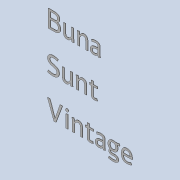
# Autodesk Inventor part: Vintage
Saved by Autodesk Inventor 2020 (Build 240168000, 168)
## iProperties
Created: 2021-01-22
Part Number: Vintage
Material: Generic
Document SubType Name: Modeling
Designer: Iulian Bors
Density: 1 g/cm^3
Appearance: Default
Author: Iulian Bors
Autodesk Inventor part; units mm, degrees
ref_plane "YZ Plane" through (0, 0, 0) normal (1, 0, 0) x (0, 1, 0)
ref_plane "XZ Plane" through (0, 0, 0) normal (0, 1, 0) x (-1, 0, 0)
ref_plane "XY Plane" through (0, 0, 0) normal (0, 0, 1) x (1, 0, 0)
sketch "Sketch1" plane through (0, 0, 0) normal (0, 0, 1) x (1, 0, 0)
  line L0 (-100, 150) -> (100, 150)
  line L1 (100, 150) -> (100, -150)
  line L2 (100, -150) -> (-100, -150)
  line L3 (-100, -150) -> (-100, 150)
  line L4 (-49.0032, 86.8855) -> (-35.0797, 86.8855) construction
  line L5 (-35.0797, 86.8855) -> (-35.0797, 72.9361) construction
  line L6 (-35.0797, 72.9361) -> (-49.0032, 72.9361) construction
  line L7 (-49.0032, 72.9361) -> (-49.0032, 86.8855) construction
  spline S0 degree 2 poles (-38.0317, 86.8855) (-36.2544, 86.8855) (-33.1501, 86.3405) (-30.8042, 84.9898) (-29.4535, 82.6675) (-29.4535, 80.8428) knots 0 0 0 1 2 3 4 4 4
  spline S1 degree 2 poles (-29.4535, 80.8428) (-29.4535, 79.7765) (-29.9511, 78.094) (-30.8279, 76.8144) (-32.1075, 75.8902) (-32.8895, 75.5822) knots 0 0 0 1 2 3 4 4 4
  line L8 (-32.8895, 75.5822) -> (-32.8895, 75.5348)
  spline S2 degree 2 poles (-32.8895, 75.5348) (-31.9416, 75.2978) (-30.1881, 74.2789) (-28.861, 72.7149) (-28.079, 70.5822) (-28.079, 69.2315) knots 0 0 0 1 2 3 4 4 4
  spline S3 degree 2 poles (-28.079, 69.2315) (-28.079, 67.2646) (-29.4772, 64.4684) (-31.9179, 62.6912) (-35.2354, 61.8618) (-37.1786, 61.8618) knots 0 0 0 1 2 3 4 4 4
  line L9 (-37.1786, 61.8618) -> (-45.899, 61.8618)
  line L10 (-45.899, 61.8618) -> (-45.899, 86.8855)
  line L11 (-45.899, 86.8855) -> (-38.0317, 86.8855)
  spline S4 degree 2 poles (-37.1786, 64.3973) (-35.9463, 64.3973) (-33.8136, 65.0135) (-32.2497, 66.2457) (-31.3492, 68.0466) (-31.3492, 69.2315) knots 0 0 0 1 2 3 4 4 4
  spline S5 degree 2 poles (-31.3492, 69.2315) (-31.3492, 70.4163) (-32.2497, 72.2172) (-33.8136, 73.4495) (-35.9463, 74.0656) (-37.1786, 74.0656) knots 0 0 0 1 2 3 4 4 4
  line L12 (-37.1786, 74.0656) -> (-42.6288, 74.0656)
  line L13 (-42.6288, 74.0656) -> (-42.6288, 64.3973)
  line L14 (-42.6288, 64.3973) -> (-37.1786, 64.3973)
  spline S6 degree 2 poles (-38.079, 76.6011) (-36.8231, 76.6011) (-34.8326, 77.0277) (-33.4819, 78.0229) (-32.7236, 79.658) (-32.7236, 80.8902) knots 0 0 0 1 2 3 4 4 4
  spline S7 degree 2 poles (-32.7236, 80.8902) (-32.7236, 81.9329) (-33.6004, 83.2836) (-34.335, 83.6627) knots 0 0 0 1 2 2 2
  spline S8 degree 2 poles (-34.335, 83.6627) (-35.0933, 84.0656) (-37.0364, 84.3499) (-38.079, 84.3499) knots 0 0 0 1 2 2 2
  line L15 (-38.079, 84.3499) -> (-42.6288, 84.3499)
  line L16 (-42.6288, 84.3499) -> (-42.6288, 76.6011)
  line L17 (-42.6288, 76.6011) -> (-38.079, 76.6011)
  line L18 (-8.5767, 62.1699) -> (-11.4677, 61.53)
  spline S9 degree 2 poles (-11.4677, 61.53) (-11.7994, 62.5727) (-11.9179, 63.5443) knots 0 0 0 1 1 1
  spline S10 degree 2 poles (-11.9179, 63.5443) (-11.989, 63.9945) (-12.1075, 65.3926) knots 0 0 0 1 1 1
  line L19 (-12.1075, 65.3926) -> (-12.4629, 65.3926)
  spline S11 degree 2 poles (-12.4629, 65.3926) (-13.4345, 63.639) (-14.8326, 62.5964) knots 0 0 0 1 1 1
  spline S12 degree 2 poles (-14.8326, 62.5964) (-16.3729, 61.4353) (-18.1027, 61.4353) knots 0 0 0 1 1 1
  spline S13 degree 2 poles (-18.1027, 61.4353) (-20.6857, 61.4353) (-22.0364, 62.6912) knots 0 0 0 1 1 1
  spline S14 degree 2 poles (-22.0364, 62.6912) (-23.1975, 63.7575) (-23.6715, 65.9376) knots 0 0 0 1 1 1
  spline S15 degree 2 poles (-23.6715, 65.9376) (-23.9558, 67.4542) (-23.9558, 70.4163) knots 0 0 0 1 1 1
  line L20 (-23.9558, 70.4163) -> (-23.9558, 79.9661)
  line L21 (-23.9558, 79.9661) -> (-20.97, 79.9661)
  line L22 (-20.97, 79.9661) -> (-20.97, 69.5632)
  spline S16 degree 2 poles (-20.97, 69.5632) (-20.97, 66.9803) (-20.4724, 65.8665) knots 0 0 0 1 1 1
  spline S17 degree 2 poles (-20.4724, 65.8665) (-19.7141, 64.2078) (-17.4629, 64.2078) knots 0 0 0 1 1 1
  spline S18 degree 2 poles (-17.4629, 64.2078) (-15.8516, 64.2078) (-14.335, 65.748) knots 0 0 0 1 1 1
  spline S19 degree 2 poles (-14.335, 65.748) (-13.2923, 66.767) (-12.1312, 68.7575) knots 0 0 0 1 1 1
  line L23 (-12.1312, 68.7575) -> (-12.1312, 79.9661)
  line L24 (-12.1312, 79.9661) -> (-9.1454, 79.9661)
  line L25 (-9.1454, 79.9661) -> (-9.1454, 68.7812)
  spline S20 degree 2 poles (-9.1454, 68.7812) (-9.1454, 66.4589) (-9.0269, 64.7528) knots 0 0 0 1 1 1
  spline S21 degree 2 poles (-9.0269, 64.7528) (-8.9558, 63.7101) (-8.5767, 62.1699) knots 0 0 0 1 1 1
  line L26 (-3.9558, 79.658) -> (-1.0885, 80.2978)
  spline S22 degree 2 poles (-1.0885, 80.2978) (-0.7568, 79.2552) (-0.6146, 78.2836) knots 0 0 0 1 1 1
  spline S23 degree 2 poles (-0.6146, 78.2836) (-0.5435, 77.8097) (-0.425, 76.4116) knots 0 0 0 1 1 1
  line L27 (-0.425, 76.4116) -> (-0.0696, 76.4116)
  spline S24 degree 2 poles (-0.0696, 76.4116) (0.8783, 78.1651) (2.3001, 79.2315) knots 0 0 0 1 1 1
  spline S25 degree 2 poles (2.3001, 79.2315) (3.8404, 80.3689) (5.5702, 80.3689) knots 0 0 0 1 1 1
  spline S26 degree 2 poles (5.5702, 80.3689) (8.1769, 80.3689) (9.5276, 79.113) knots 0 0 0 1 1 1
  spline S27 degree 2 poles (9.5276, 79.113) (10.6887, 78.0466) (11.1627, 75.8665) knots 0 0 0 1 1 1
  spline S28 degree 2 poles (11.1627, 75.8665) (11.447, 74.3736) (11.447, 71.4116) knots 0 0 0 1 1 1
  line L28 (11.447, 71.4116) -> (11.447, 61.8618)
  line L29 (11.447, 61.8618) -> (8.4612, 61.8618)
  line L30 (8.4612, 61.8618) -> (8.4612, 72.2409)
  spline S29 degree 2 poles (8.4612, 72.2409) (8.4612, 74.8239) (7.9636, 75.9376) knots 0 0 0 1 1 1
  spline S30 degree 2 poles (7.9636, 75.9376) (7.2053, 77.5964) (4.9304, 77.5964) knots 0 0 0 1 1 1
  spline S31 degree 2 poles (4.9304, 77.5964) (3.3428, 77.5964) (1.8025, 76.0561) knots 0 0 0 1 1 1
  spline S32 degree 2 poles (1.8025, 76.0561) (0.7598, 75.0371) (-0.4013, 73.0466) knots 0 0 0 1 1 1
  line L31 (-0.4013, 73.0466) -> (-0.4013, 61.8618)
  line L32 (-0.4013, 61.8618) -> (-3.3871, 61.8618)
  line L33 (-3.3871, 61.8618) -> (-3.3871, 72.9992)
  spline S33 degree 2 poles (-3.3871, 72.9992) (-3.3871, 75.3452) (-3.5056, 77.0514) knots 0 0 0 1 1 1
  spline S34 degree 2 poles (-3.5056, 77.0514) (-3.5767, 78.1177) (-3.9558, 79.658) knots 0 0 0 1 1 1
  line L34 (17.6319, 76.767) -> (16.8736, 79.2078)
  spline S35 degree 2 poles (16.8736, 79.2078) (19.7883, 80.3689) (22.9873, 80.3689) knots 0 0 0 1 1 1
  spline S36 degree 2 poles (22.9873, 80.3689) (25.7835, 80.3689) (27.2764, 79.421) knots 0 0 0 1 1 1
  spline S37 degree 2 poles (27.2764, 79.421) (28.9589, 78.3547) (28.9589, 75.748) knots 0 0 0 1 1 1
  line L35 (28.9589, 75.748) -> (28.9589, 68.639)
  spline S38 degree 2 poles (28.9589, 68.639) (28.9589, 67.1935) (28.9826, 65.7007) knots 0 0 0 1 1 1
  spline S39 degree 2 poles (28.9826, 65.7007) (29.0063, 64.8239) (29.1721, 63.8523) knots 0 0 0 1 1 1
  spline S40 degree 2 poles (29.1721, 63.8523) (29.2906, 62.9518) (29.5276, 62.1225) knots 0 0 0 1 1 1
  line L36 (29.5276, 62.1225) -> (26.684, 61.5063)
  spline S41 degree 2 poles (26.684, 61.5063) (26.2811, 62.6675) (26.1627, 64.113) knots 0 0 0 1 1 1
  line L37 (26.1627, 64.113) -> (25.8309, 64.1604)
  spline S42 degree 2 poles (25.8309, 64.1604) (23.6745, 61.4353) (20.3333, 61.4353) knots 0 0 0 1 1 1
  spline S43 degree 2 poles (20.3333, 61.4353) (17.8925, 61.4353) (14.9304, 64.1367) (14.9304, 66.6011) knots 0 0 0 1 2 2 2
  spline S44 degree 2 poles (14.9304, 66.6011) (14.9304, 68.4258) (16.5418, 70.7717) (18.0347, 71.5537) knots 0 0 0 1 2 2 2
  spline S45 degree 2 poles (18.0347, 71.5537) (20.357, 72.8334) (24.5513, 72.8334) knots 0 0 0 1 1 1
  spline S46 degree 2 poles (24.5513, 72.8334) (25.12, 72.8334) (26.0442, 72.8097) knots 0 0 0 1 1 1
  line L38 (26.0442, 72.8097) -> (26.0442, 75.44)
  spline S47 degree 2 poles (26.0442, 75.44) (26.0442, 76.6959) (24.5276, 77.8097) (22.8925, 77.8097) knots 0 0 0 1 2 2 2
  spline S48 degree 2 poles (22.8925, 77.8097) (20.4992, 77.8097) (17.6319, 76.767) knots 0 0 0 1 1 1
  line L39 (26.0442, 66.9329) -> (26.0442, 70.6059)
  spline S49 degree 2 poles (26.0442, 70.6059) (25.5702, 70.6296) (24.6698, 70.6296) knots 0 0 0 1 1 1
  spline S50 degree 2 poles (24.6698, 70.6296) (23.1532, 70.6296) (21.8499, 70.3689) knots 0 0 0 1 1 1
  spline S51 degree 2 poles (21.8499, 70.3689) (19.9541, 69.9898) (17.8451, 68.331) (17.8451, 66.7907) knots 0 0 0 1 2 2 2
  spline S52 degree 2 poles (17.8451, 66.7907) (17.8451, 63.9945) (20.8783, 63.9945) knots 0 0 0 1 1 1
  spline S53 degree 2 poles (20.8783, 63.9945) (22.4423, 63.9945) (23.793, 64.8239) knots 0 0 0 1 1 1
  spline S54 degree 2 poles (23.793, 64.8239) (24.9067, 65.5348) (26.0442, 66.9329) knots 0 0 0 1 1 1
  spline S55 degree 2 poles (-45.97, 9.0243) (-45.2591, 8.74) (-43.6715, 8.2661) (-42.0127, 7.9106) (-40.3539, 7.6973) (-39.5482, 7.6973) knots 0 0 0 1 2 3 4 4 4
  spline S56 degree 2 poles (-39.5482, 7.6973) (-38.1738, 7.6973) (-35.9463, 8.3134) (-34.3587, 9.522) (-33.4819, 11.2755) (-33.4819, 12.413) knots 0 0 0 1 2 3 4 4 4
  spline S57 degree 2 poles (-33.4819, 12.413) (-33.4819, 13.5504) (-34.2876, 14.9959) (-35.8279, 15.9675) (-38.1027, 16.6547) (-39.5482, 17.0101) knots 0 0 0 1 2 3 4 4 4
  spline S58 degree 2 poles (-39.5482, 17.0101) (-41.1596, 17.413) (-43.8373, 18.4556) (-45.8042, 20.0907) (-46.9179, 22.5078) (-46.9179, 24.3324) knots 0 0 0 1 2 3 4 4 4
  spline S59 degree 2 poles (-46.9179, 24.3324) (-46.9179, 25.8016) (-45.7331, 28.195) (-43.5767, 29.9011) (-40.5672, 30.8016) (-38.7189, 30.8016) knots 0 0 0 1 2 3 4 4 4
  spline S60 degree 2 poles (-38.7189, 30.8016) (-37.8421, 30.8016) (-35.9937, 30.5646) (-34.1928, 30.1855) (-32.4392, 29.6405) (-31.6809, 29.3087) knots 0 0 0 1 2 3 4 4 4
  line L40 (-31.6809, 29.3087) -> (-32.7236, 26.7258)
  spline S61 degree 2 poles (-32.7236, 26.7258) (-33.3634, 26.9864) (-34.6667, 27.4604) (-36.1122, 27.8395) (-37.771, 28.0765) (-38.7189, 28.0765) knots 0 0 0 1 2 3 4 4 4
  spline S62 degree 2 poles (-38.7189, 28.0765) (-39.6904, 28.0765) (-41.4203, 27.6499) (-42.771, 26.7732) (-43.553, 25.3514) (-43.553, 24.3324) knots 0 0 0 1 2 3 4 4 4
  spline S63 degree 2 poles (-43.553, 24.3324) (-43.553, 23.195) (-42.7473, 21.7495) (-41.207, 20.7779) (-38.9321, 20.0907) (-37.4866, 19.7352) knots 0 0 0 1 2 3 4 4 4
  spline S64 degree 2 poles (-37.4866, 19.7352) (-35.899, 19.3087) (-33.1975, 18.2898) (-31.2307, 16.6547) (-30.117, 14.2139) (-30.117, 12.413) knots 0 0 0 1 2 3 4 4 4
  spline S65 degree 2 poles (-30.117, 12.413) (-30.117, 10.5172) (-31.5151, 7.721) (-34.0506, 5.8727) (-37.5103, 4.9722) (-39.5482, 4.9722) knots 0 0 0 1 2 3 4 4 4
  spline S66 degree 2 poles (-39.5482, 4.9722) (-43.3871, 4.9722) (-47.0127, 6.4414) knots 0 0 0 1 1 1
  line L41 (-47.0127, 6.4414) -> (-45.97, 9.0243)
  line L42 (-10.3302, 5.7068) -> (-13.2212, 5.067)
  spline S67 degree 2 poles (-13.2212, 5.067) (-13.553, 6.1097) (-13.6715, 7.0812) knots 0 0 0 1 1 1
  spline S68 degree 2 poles (-13.6715, 7.0812) (-13.7426, 7.5315) (-13.861, 8.9296) knots 0 0 0 1 1 1
  line L43 (-13.861, 8.9296) -> (-14.2165, 8.9296)
  spline S69 degree 2 poles (-14.2165, 8.9296) (-15.1881, 7.176) (-16.5862, 6.1334) knots 0 0 0 1 1 1
  spline S70 degree 2 poles (-16.5862, 6.1334) (-18.1264, 4.9722) (-19.8563, 4.9722) knots 0 0 0 1 1 1
  spline S71 degree 2 poles (-19.8563, 4.9722) (-22.4392, 4.9722) (-23.7899, 6.2281) knots 0 0 0 1 1 1
  spline S72 degree 2 poles (-23.7899, 6.2281) (-24.9511, 7.2945) (-25.425, 9.4746) knots 0 0 0 1 1 1
  spline S73 degree 2 poles (-25.425, 9.4746) (-25.7094, 10.9912) (-25.7094, 13.9533) knots 0 0 0 1 1 1
  line L44 (-25.7094, 13.9533) -> (-25.7094, 23.503)
  line L45 (-25.7094, 23.503) -> (-22.7236, 23.503)
  line L46 (-22.7236, 23.503) -> (-22.7236, 13.1002)
  spline S74 degree 2 poles (-22.7236, 13.1002) (-22.7236, 10.5172) (-22.226, 9.4035) knots 0 0 0 1 1 1
  spline S75 degree 2 poles (-22.226, 9.4035) (-21.4677, 7.7447) (-19.2165, 7.7447) knots 0 0 0 1 1 1
  spline S76 degree 2 poles (-19.2165, 7.7447) (-17.6051, 7.7447) (-16.0885, 9.285) knots 0 0 0 1 1 1
  spline S77 degree 2 poles (-16.0885, 9.285) (-15.0459, 10.304) (-13.8847, 12.2945) knots 0 0 0 1 1 1
  line L47 (-13.8847, 12.2945) -> (-13.8847, 23.503)
  line L48 (-13.8847, 23.503) -> (-10.899, 23.503)
  line L49 (-10.899, 23.503) -> (-10.899, 12.3182)
  spline S78 degree 2 poles (-10.899, 12.3182) (-10.899, 9.9959) (-10.7805, 8.2898) knots 0 0 0 1 1 1
  spline S79 degree 2 poles (-10.7805, 8.2898) (-10.7094, 7.2471) (-10.3302, 5.7068) knots 0 0 0 1 1 1
  line L50 (-5.7094, 23.195) -> (-2.8421, 23.8348)
  spline S80 degree 2 poles (-2.8421, 23.8348) (-2.5103, 22.7921) (-2.3681, 21.8206) knots 0 0 0 1 1 1
  spline S81 degree 2 poles (-2.3681, 21.8206) (-2.2971, 21.3466) (-2.1786, 19.9485) knots 0 0 0 1 1 1
  line L51 (-2.1786, 19.9485) -> (-1.8231, 19.9485)
  spline S82 degree 2 poles (-1.8231, 19.9485) (-0.8753, 21.7021) (0.5465, 22.7684) knots 0 0 0 1 1 1
  spline S83 degree 2 poles (0.5465, 22.7684) (2.0868, 23.9059) (3.8167, 23.9059) knots 0 0 0 1 1 1
  spline S84 degree 2 poles (3.8167, 23.9059) (6.4233, 23.9059) (7.774, 22.6499) knots 0 0 0 1 1 1
  spline S85 degree 2 poles (7.774, 22.6499) (8.9352, 21.5836) (9.4091, 19.4035) knots 0 0 0 1 1 1
  spline S86 degree 2 poles (9.4091, 19.4035) (9.6935, 17.9106) (9.6935, 14.9485) knots 0 0 0 1 1 1
  line L52 (9.6935, 14.9485) -> (9.6935, 5.3988)
  line L53 (9.6935, 5.3988) -> (6.7077, 5.3988)
  line L54 (6.7077, 5.3988) -> (6.7077, 15.7779)
  spline S87 degree 2 poles (6.7077, 15.7779) (6.7077, 18.3608) (6.2101, 19.4746) knots 0 0 0 1 1 1
  spline S88 degree 2 poles (6.2101, 19.4746) (5.4518, 21.1334) (3.1769, 21.1334) knots 0 0 0 1 1 1
  spline S89 degree 2 poles (3.1769, 21.1334) (1.5892, 21.1334) (0.0489, 19.5931) knots 0 0 0 1 1 1
  spline S90 degree 2 poles (0.0489, 19.5931) (-0.9937, 18.5741) (-2.1549, 16.5836) knots 0 0 0 1 1 1
  line L55 (-2.1549, 16.5836) -> (-2.1549, 5.3988)
  line L56 (-2.1549, 5.3988) -> (-5.1407, 5.3988)
  line L57 (-5.1407, 5.3988) -> (-5.1407, 16.5362)
  spline S91 degree 2 poles (-5.1407, 16.5362) (-5.1407, 18.8822) (-5.2591, 20.5883) knots 0 0 0 1 1 1
  spline S92 degree 2 poles (-5.2591, 20.5883) (-5.3302, 21.6547) (-5.7094, 23.195) knots 0 0 0 1 1 1
  line L58 (16.4233, 27.6499) -> (19.4091, 27.6499)
  line L59 (19.4091, 27.6499) -> (19.4091, 23.503)
  line L60 (19.4091, 23.503) -> (25.4992, 23.503)
  line L61 (25.4992, 23.503) -> (25.4992, 20.9912)
  line L62 (25.4992, 20.9912) -> (19.4091, 20.9912)
  line L63 (19.4091, 20.9912) -> (19.4091, 10.5646)
  spline S93 degree 2 poles (19.4091, 10.5646) (19.4091, 9.522) (19.5276, 8.4319) (19.7646, 8.1239) knots 0 0 0 1 2 2 2
  spline S94 degree 2 poles (19.7646, 8.1239) (20.2385, 7.4841) (21.6129, 7.4841) knots 0 0 0 1 1 1
  spline S95 degree 2 poles (21.6129, 7.4841) (22.3712, 7.4841) (23.0821, 7.6499) knots 0 0 0 1 1 1
  spline S96 degree 2 poles (23.0821, 7.6499) (23.8167, 7.7921) (24.4328, 7.9817) knots 0 0 0 1 1 1
  spline S97 degree 2 poles (24.4328, 7.9817) (24.9067, 6.939) (25.3096, 5.6594) knots 0 0 0 1 1 1
  spline S98 degree 2 poles (25.3096, 5.6594) (23.248, 4.9722) (21.1627, 4.9722) knots 0 0 0 1 1 1
  spline S99 degree 2 poles (21.1627, 4.9722) (19.6698, 4.9722) (17.8214, 5.6594) (17.3001, 6.4177) knots 0 0 0 1 2 2 2
  spline S100 degree 2 poles (17.3001, 6.4177) (16.7788, 7.2234) (16.4233, 9.4509) (16.4233, 11.4177) knots 0 0 0 1 2 2 2
  line L64 (16.4233, 11.4177) -> (16.4233, 20.9912)
  line L65 (16.4233, 20.9912) -> (13.8167, 20.9912)
  line L66 (13.8167, 20.9912) -> (13.8167, 23.503)
  line L67 (13.8167, 23.503) -> (16.4233, 23.503)
  line L68 (16.4233, 23.503) -> (16.4233, 27.6499)
  line L69 (-28.861, -26.0406) -> (-25.425, -26.0406)
  line L70 (-25.425, -26.0406) -> (-34.7615, -51.088)
  line L71 (-34.7615, -51.088) -> (-37.6762, -51.088)
  line L72 (-37.6762, -51.088) -> (-47.0364, -26.0406)
  line L73 (-47.0364, -26.0406) -> (-43.6004, -26.0406)
  line L74 (-43.6004, -26.0406) -> (-36.207, -47.0595)
  line L75 (-36.207, -47.0595) -> (-28.861, -26.0406)
  line L76 (-20.3065, -32.96) -> (-17.3208, -32.96)
  line L77 (-17.3208, -32.96) -> (-17.3208, -51.0643)
  line L78 (-17.3208, -51.0643) -> (-20.3065, -51.0643)
  line L79 (-20.3065, -51.0643) -> (-20.3065, -32.96)
  spline S101 degree 2 poles (-18.7899, -25.9458) (-17.9843, -25.9458) (-17.3918, -26.4908) knots 0 0 0 1 1 1
  spline S102 degree 2 poles (-17.3918, -26.4908) (-16.8231, -27.1069) (-16.8231, -27.9363) knots 0 0 0 1 1 1
  spline S103 degree 2 poles (-16.8231, -27.9363) (-16.8231, -28.7657) (-17.3918, -29.3344) knots 0 0 0 1 1 1
  spline S104 degree 2 poles (-17.3918, -29.3344) (-17.9843, -29.9268) (-18.7899, -29.9268) knots 0 0 0 1 1 1
  spline S105 degree 2 poles (-18.7899, -29.9268) (-19.6193, -29.9268) (-20.2117, -29.3344) knots 0 0 0 1 1 1
  spline S106 degree 2 poles (-20.2117, -29.3344) (-20.8042, -28.7894) (-20.8042, -27.9363) knots 0 0 0 1 1 1
  spline S107 degree 2 poles (-20.8042, -27.9363) (-20.8042, -27.0832) (-20.2117, -26.4908) knots 0 0 0 1 1 1
  spline S108 degree 2 poles (-20.2117, -26.4908) (-19.6193, -25.9458) (-18.7899, -25.9458) knots 0 0 0 1 1 1
  line L80 (-11.6572, -33.2681) -> (-8.7899, -32.6283)
  spline S109 degree 2 poles (-8.7899, -32.6283) (-8.4582, -33.6709) (-8.316, -34.6425) knots 0 0 0 1 1 1
  spline S110 degree 2 poles (-8.316, -34.6425) (-8.2449, -35.1164) (-8.1264, -36.5145) knots 0 0 0 1 1 1
  line L81 (-8.1264, -36.5145) -> (-7.771, -36.5145)
  spline S111 degree 2 poles (-7.771, -36.5145) (-6.8231, -34.761) (-5.4013, -33.6946) knots 0 0 0 1 1 1
  spline S112 degree 2 poles (-5.4013, -33.6946) (-3.861, -32.5572) (-2.1312, -32.5572) knots 0 0 0 1 1 1
  spline S113 degree 2 poles (-2.1312, -32.5572) (0.4755, -32.5572) (1.8262, -33.8131) knots 0 0 0 1 1 1
  spline S114 degree 2 poles (1.8262, -33.8131) (2.9873, -34.8794) (3.4612, -37.0595) knots 0 0 0 1 1 1
  spline S115 degree 2 poles (3.4612, -37.0595) (3.7456, -38.5524) (3.7456, -41.5145) knots 0 0 0 1 1 1
  line L82 (3.7456, -41.5145) -> (3.7456, -51.0643)
  line L83 (3.7456, -51.0643) -> (0.7598, -51.0643)
  line L84 (0.7598, -51.0643) -> (0.7598, -40.6851)
  spline S116 degree 2 poles (0.7598, -40.6851) (0.7598, -38.1022) (0.2622, -36.9885) knots 0 0 0 1 1 1
  spline S117 degree 2 poles (0.2622, -36.9885) (-0.4961, -35.3297) (-2.771, -35.3297) knots 0 0 0 1 1 1
  spline S118 degree 2 poles (-2.771, -35.3297) (-4.3587, -35.3297) (-5.899, -36.87) knots 0 0 0 1 1 1
  spline S119 degree 2 poles (-5.899, -36.87) (-6.9416, -37.8889) (-8.1027, -39.8794) knots 0 0 0 1 1 1
  line L85 (-8.1027, -39.8794) -> (-8.1027, -51.0643)
  line L86 (-8.1027, -51.0643) -> (-11.0885, -51.0643)
  line L87 (-11.0885, -51.0643) -> (-11.0885, -39.9268)
  spline S120 degree 2 poles (-11.0885, -39.9268) (-11.0885, -37.5809) (-11.207, -35.8747) knots 0 0 0 1 1 1
  spline S121 degree 2 poles (-11.207, -35.8747) (-11.2781, -34.8084) (-11.6572, -33.2681) knots 0 0 0 1 1 1
  line L88 (10.4755, -28.8131) -> (13.4612, -28.8131)
  line L89 (13.4612, -28.8131) -> (13.4612, -32.96)
  line L90 (13.4612, -32.96) -> (19.5513, -32.96)
  line L91 (19.5513, -32.96) -> (19.5513, -35.4719)
  line L92 (19.5513, -35.4719) -> (13.4612, -35.4719)
  line L93 (13.4612, -35.4719) -> (13.4612, -45.8984)
  spline S122 degree 2 poles (13.4612, -45.8984) (13.4612, -46.9411) (13.5797, -48.0311) (13.8167, -48.3392) knots 0 0 0 1 2 2 2
  spline S123 degree 2 poles (13.8167, -48.3392) (14.2906, -48.979) (15.665, -48.979) knots 0 0 0 1 1 1
  spline S124 degree 2 poles (15.665, -48.979) (16.4233, -48.979) (17.1342, -48.8131) knots 0 0 0 1 1 1
  spline S125 degree 2 poles (17.1342, -48.8131) (17.8688, -48.6709) (18.4849, -48.4813) knots 0 0 0 1 1 1
  spline S126 degree 2 poles (18.4849, -48.4813) (18.9589, -49.524) (19.3617, -50.8036) knots 0 0 0 1 1 1
  spline S127 degree 2 poles (19.3617, -50.8036) (17.3001, -51.4908) (15.2148, -51.4908) knots 0 0 0 1 1 1
  spline S128 degree 2 poles (15.2148, -51.4908) (13.7219, -51.4908) (11.8736, -50.8036) (11.3522, -50.0453) knots 0 0 0 1 2 2 2
  spline S129 degree 2 poles (11.3522, -50.0453) (10.8309, -49.2396) (10.4755, -47.0121) (10.4755, -45.0453) knots 0 0 0 1 2 2 2
  line L94 (10.4755, -45.0453) -> (10.4755, -35.4719)
  line L95 (10.4755, -35.4719) -> (7.8688, -35.4719)
  line L96 (7.8688, -35.4719) -> (7.8688, -32.96)
  line L97 (7.8688, -32.96) -> (10.4755, -32.96)
  line L98 (10.4755, -32.96) -> (10.4755, -28.8131)
  line L99 (24.9067, -36.1591) -> (24.1484, -33.7183)
  spline S130 degree 2 poles (24.1484, -33.7183) (27.0631, -32.5572) (30.2622, -32.5572) knots 0 0 0 1 1 1
  spline S131 degree 2 poles (30.2622, -32.5572) (33.0584, -32.5572) (34.5513, -33.505) knots 0 0 0 1 1 1
  spline S132 degree 2 poles (34.5513, -33.505) (36.2337, -34.5714) (36.2337, -37.178) knots 0 0 0 1 1 1
  line L100 (36.2337, -37.178) -> (36.2337, -44.287)
  spline S133 degree 2 poles (36.2337, -44.287) (36.2337, -45.7325) (36.2574, -47.2254) knots 0 0 0 1 1 1
  spline S134 degree 2 poles (36.2574, -47.2254) (36.2811, -48.1022) (36.447, -49.0738) knots 0 0 0 1 1 1
  spline S135 degree 2 poles (36.447, -49.0738) (36.5655, -49.9742) (36.8025, -50.8036) knots 0 0 0 1 1 1
  line L101 (36.8025, -50.8036) -> (33.9589, -51.4197)
  spline S136 degree 2 poles (33.9589, -51.4197) (33.556, -50.2586) (33.4375, -48.8131) knots 0 0 0 1 1 1
  line L102 (33.4375, -48.8131) -> (33.1058, -48.7657)
  spline S137 degree 2 poles (33.1058, -48.7657) (30.9494, -51.4908) (27.6082, -51.4908) knots 0 0 0 1 1 1
  spline S138 degree 2 poles (27.6082, -51.4908) (25.1674, -51.4908) (22.2053, -48.7894) (22.2053, -46.3249) knots 0 0 0 1 2 2 2
  spline S139 degree 2 poles (22.2053, -46.3249) (22.2053, -44.5003) (23.8167, -42.1543) (25.3096, -41.3723) knots 0 0 0 1 2 2 2
  spline S140 degree 2 poles (25.3096, -41.3723) (27.6319, -40.0927) (31.8262, -40.0927) knots 0 0 0 1 1 1
  spline S141 degree 2 poles (31.8262, -40.0927) (32.3949, -40.0927) (33.3191, -40.1164) knots 0 0 0 1 1 1
  line L103 (33.3191, -40.1164) -> (33.3191, -37.4861)
  spline S142 degree 2 poles (33.3191, -37.4861) (33.3191, -36.2302) (31.8025, -35.1164) (30.1674, -35.1164) knots 0 0 0 1 2 2 2
  spline S143 degree 2 poles (30.1674, -35.1164) (27.774, -35.1164) (24.9067, -36.1591) knots 0 0 0 1 1 1
  line L104 (33.3191, -45.9932) -> (33.3191, -42.3202)
  spline S144 degree 2 poles (33.3191, -42.3202) (32.8451, -42.2965) (31.9446, -42.2965) knots 0 0 0 1 1 1
  spline S145 degree 2 poles (31.9446, -42.2965) (30.4281, -42.2965) (29.1247, -42.5572) knots 0 0 0 1 1 1
  spline S146 degree 2 poles (29.1247, -42.5572) (27.229, -42.9363) (25.12, -44.5951) (25.12, -46.1354) knots 0 0 0 1 2 2 2
  spline S147 degree 2 poles (25.12, -46.1354) (25.12, -48.9316) (28.1532, -48.9316) knots 0 0 0 1 1 1
  spline S148 degree 2 poles (28.1532, -48.9316) (29.7172, -48.9316) (31.0679, -48.1022) knots 0 0 0 1 1 1
  spline S149 degree 2 poles (31.0679, -48.1022) (32.1816, -47.3913) (33.3191, -45.9932) knots 0 0 0 1 1 1
  spline S150 degree 2 poles (52.3001, -32.96) (53.0347, -32.96) (54.1721, -32.9126) (55.2148, -32.7941) (56.2811, -32.5572) (56.992, -32.3202) knots 0 0 0 1 2 3 4 4 4
  spline S151 degree 2 poles (56.992, -32.3202) (57.229, -32.9837) (57.6555, -34.1685) (57.8688, -34.7847) knots 0 0 0 1 2 2 2
  spline S152 degree 2 poles (57.8688, -34.7847) (57.3238, -34.9979) (56.3759, -35.2586) (55.4518, -35.4008) (54.5276, -35.4482) (54.0063, -35.4719) knots 0 0 0 1 2 3 4 4 4
  spline S153 degree 2 poles (54.0063, -35.4719) (54.5039, -36.2539) (55.0252, -38.2207) (55.0252, -39.3581) knots 0 0 0 1 2 2 2
  spline S154 degree 2 poles (55.0252, -39.3581) (55.0252, -41.0406) (54.0063, -43.5287) (53.0821, -44.4055) knots 0 0 0 1 2 2 2
  spline S155 degree 2 poles (53.0821, -44.4055) (52.1342, -45.2586) (49.5039, -46.1591) (47.8688, -46.1591) knots 0 0 0 1 2 2 2
  spline S156 degree 2 poles (47.8688, -46.1591) (47.0394, -46.1591) (45.5465, -45.9695) (44.8593, -45.7325) knots 0 0 0 1 2 2 2
  spline S157 degree 2 poles (44.8593, -45.7325) (44.7172, -46.1354) (44.4802, -47.0121) (44.5039, -47.7941) (44.7646, -48.4339) (45.12, -48.6472) knots 0 0 0 1 2 3 4 4 4
  spline S158 degree 2 poles (45.12, -48.6472) (45.2859, -48.742) (45.6887, -48.8605) (46.2101, -48.9553) (46.992, -49.0027) (47.5134, -49.0027) knots 0 0 0 1 2 3 4 4 4
  spline S159 degree 2 poles (47.5134, -49.0027) (48.0584, -49.0264) (49.4565, -49.0264) (50.4044, -49.0264) knots 0 0 0 1 2 2 2
  spline S160 degree 2 poles (50.4044, -49.0264) (53.1058, -49.0264) (55.902, -51.3012) (55.902, -53.6946) knots 0 0 0 1 2 2 2
  spline S161 degree 2 poles (55.902, -53.6946) (55.902, -54.6662) (55.2622, -56.1828) (54.1721, -57.2965) (52.6792, -58.0311) (50.9257, -58.505) (49.03, -58.6946) (48.0821, -58.6946) knots 0 0 0 1 2 3 4 5 6 6 6
  spline S162 degree 2 poles (48.0821, -58.6946) (47.1105, -58.6946) (45.1911, -58.4813) (44.2669, -58.3392) knots 0 0 0 1 2 2 2
  spline S163 degree 2 poles (44.2669, -58.3392) (43.3428, -58.1733) (41.7314, -57.7704) (41.0916, -57.5809) knots 0 0 0 1 2 2 2
  spline S164 degree 2 poles (41.0916, -57.5809) (41.3285, -56.9885) (41.9446, -55.8036) (42.3001, -55.2823) knots 0 0 0 1 2 2 2
  spline S165 degree 2 poles (42.3001, -55.2823) (43.3901, -55.5903) (46.4233, -56.1828) (48.2717, -56.1828) knots 0 0 0 1 2 2 2
  spline S166 degree 2 poles (48.2717, -56.1828) (49.101, -56.1828) (50.7361, -55.9695) (52.0394, -55.4008) (52.8451, -54.4529) (52.8451, -53.6946) knots 0 0 0 1 2 3 4 4 4
  spline S167 degree 2 poles (52.8451, -53.6946) (52.8451, -52.8889) (52.2527, -52.0121) (51.2811, -51.6093) (49.9541, -51.5382) (49.2432, -51.5382) knots 0 0 0 1 2 3 4 4 4
  line L105 (49.2432, -51.5382) -> (46.9446, -51.5382)
  spline S168 degree 2 poles (46.9446, -51.5382) (45.9257, -51.5382) (44.101, -51.2302) (42.7503, -50.4719) (41.9683, -49.2633) (41.9683, -48.3629) knots 0 0 0 1 2 3 4 4 4
  spline S169 degree 2 poles (41.9683, -48.3629) (41.9683, -47.5098) (42.5845, -45.6851) (43.1058, -44.7373) knots 0 0 0 1 2 2 2
  spline S170 degree 2 poles (43.1058, -44.7373) (41.9446, -43.9079) (40.7124, -41.1591) (40.7124, -39.3581) knots 0 0 0 1 2 2 2
  spline S171 degree 2 poles (40.7124, -39.3581) (40.7124, -37.723) (41.7314, -35.2112) (42.6792, -34.3107) knots 0 0 0 1 2 2 2
  spline S172 degree 2 poles (42.6792, -34.3107) (43.6271, -33.4339) (46.2337, -32.5572) (47.8688, -32.5572) knots 0 0 0 1 2 2 2
  spline S173 degree 2 poles (47.8688, -32.5572) (49.4091, -32.5572) (50.6887, -32.96) knots 0 0 0 1 1 1
  line L106 (50.6887, -32.96) -> (52.3001, -32.96)
  spline S174 degree 2 poles (47.8688, -34.9505) (46.7788, -34.9505) (45.2148, -35.614) (44.2195, -36.7752) (43.7456, -38.4103) (43.7456, -39.3581) knots 0 0 0 1 2 3 4 4 4
  spline S175 degree 2 poles (43.7456, -39.3581) (43.7456, -40.3534) (44.2195, -41.9411) (45.2148, -43.1259) (46.7788, -43.7657) (47.8688, -43.7657) knots 0 0 0 1 2 3 4 4 4
  spline S176 degree 2 poles (47.8688, -43.7657) (48.9589, -43.7657) (50.5228, -43.1259) (51.5181, -41.9411) (51.992, -40.3297) (51.992, -39.3581) knots 0 0 0 1 2 3 4 4 4
  spline S177 degree 2 poles (51.992, -39.3581) (51.992, -38.4103) (51.5181, -36.7752) (50.5228, -35.614) (48.9589, -34.9505) (47.8688, -34.9505) knots 0 0 0 1 2 3 4 4 4
  spline S178 degree 2 poles (74.9541, -50.069) (73.011, -50.8273) (69.6224, -51.4908) (68.2717, -51.4908) knots 0 0 0 1 2 2 2
  spline S179 degree 2 poles (68.2717, -51.4908) (66.2337, -51.4908) (63.1532, -50.1875) (61.1153, -47.8178) (60.0963, -44.524) (60.0963, -42.5335) knots 0 0 0 1 2 3 4 4 4
  spline S180 degree 2 poles (60.0963, -42.5335) (60.0963, -41.3249) (60.4518, -38.8842) (61.2101, -36.6567) (62.4423, -34.761) (64.2195, -33.3629) (66.5892, -32.5572) (68.1058, -32.5572) knots 0 0 0 1 2 3 4 5 6 6 6
  spline S181 degree 2 poles (68.1058, -32.5572) (71.992, -32.5572) (75.9257, -37.415) (75.9257, -41.9648) knots 0 0 0 1 2 2 2
  line L107 (75.9257, -41.9648) -> (75.9257, -42.9126)
  line L108 (75.9257, -42.9126) -> (63.1769, -42.9126)
  spline S182 degree 2 poles (63.1769, -42.9126) (63.1769, -44.3818) (63.793, -46.633) (65.12, -48.1733) (67.1105, -48.979) (68.4849, -48.979) knots 0 0 0 1 2 3 4 4 4
  spline S183 degree 2 poles (68.4849, -48.979) (69.2669, -48.979) (70.7835, -48.742) (72.2053, -48.3866) (73.5086, -47.9363) (74.0773, -47.723) knots 0 0 0 1 2 3 4 4 4
  line L109 (74.0773, -47.723) -> (74.9541, -50.069)
  spline S184 degree 2 poles (72.9162, -40.5193) (72.774, -37.6757) (70.357, -35.069) (68.1058, -35.069) knots 0 0 0 1 2 2 2
  spline S185 degree 2 poles (68.1058, -35.069) (65.8546, -35.069) (63.5086, -37.6757) (63.2717, -40.5193) knots 0 0 0 1 2 2 2
  line L110 (63.2717, -40.5193) -> (72.9162, -40.5193)
  point P0 (0, 0)
  point P1 (0, 150)
  point P2 (-100, 0)
  dimension "d0" = 300
  dimension "d1" = 200
  constraints: 8 end point, 2 midpoint, 2 parallel, 1 horizontal, 1 horizontal alignment, 1 perpendicular, 1 vertical alignment, 2 other
  measures "d0" distance of L2.end L0.start
  measures "d1" distance of L1.end L2.end
extrude "Extrusion1" add sketch "Sketch1" along normal blind 0.6 contours S0 S1 L8 S2 S3 L9 L10 L11 | L18 S9 S10 L19 S11 S12 S13 S14 S15 L20 L21 L22 S16 S17 S18 S19 L23 L24 L25 S20 S21 | L26 S22 S23 L27 S24 S25 S26 S27 S28 L28 L29 L30 S29 S30 S31 S32 L31 L32 L33 S33 S34 | L34 S35 S36 S37 L35 S38 S39 S40 L36 S41 L37 S42 S43 S44 S45 S46 L38 S47 S48 | S55 S56 S57 S58 S59 S60 L40 S61 S62 S63 S64 S65 S66 L41 | L42 S67 S68 L43 S69 S70 S71 S72 S73 L44 L45 L46 S74 S75 S76 S77 L47 L48 L49 S78 S79 | L50 S80 S81 L51 S82 S83 S84 S85 S86 L52 L53 L54 S87 S88 S89 S90 L55 L56 L57 S91 S92 | L58 L59 L60 L61 L62 L63 S93 S94 S95 S96 S97 S98 S99 S100 L64 L65 L66 L67 L68 | L69 L70 L71 L72 L73 L74 L75 | L76 L77 L78 L79 | S101 S102 S103 S104 S105 S106 S107 S108 | L80 S109 S110 L81 S111 S112 S113 S114 S115 L82 L83 L84 S116 S117 S118 S119 L85 L86 L87 S120 S121 | L88 L89 L90 L91 L92 L93 S122 S123 S124 S125 S126 S127 S128 S129 L94 L95 L96 L97 L98 | L99 S130 S131 S132 L100 S133 S134 S135 L101 S136 L102 S137 S138 S139 S140 S141 L103 S142 S143 | S150 S151 S152 S153 S154 S155 S156 S157 S158 S159 S160 S161 S162 S163 S164 S165 S166 S167 L105 S168 S169 S170 S171 S172 S173 L106 | S178 S179 S180 S181 L107 L108 S182 S183 L109
body "Solid1"
